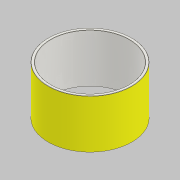
# Autodesk Inventor part: Stator Metal Ring
Saved by Autodesk Inventor 2020.1 (Build 241239000, 239)
## iProperties
Created: 2019-08-27
Part Number: Stator Metal Ring
Material: Steel, Wrought
Document SubType Name: Modeling
Designer: Oliver Frolovs
Density: 7.85 g/cm^3
Appearance: Steel
Mass: 2564.86 g
Surface Area: 1199.24 cm^2
Volume: 326.733 cm^3
Author: Oliver Frolovs
Autodesk Inventor part; units mm, degrees
ref_plane "YZ Plane" through (0, 0, 0) normal (1, 0, 0) x (0, 1, 0)
ref_plane "XZ Plane" through (0, 0, 0) normal (0, 1, 0) x (-1, 0, 0)
ref_plane "XY Plane" through (0, 0, 0) normal (0, 0, 1) x (1, 0, 0)
sketch "Sketch Metal Ring Profile" plane through (0, 0, 0) normal (0, 0, 1) x (1, 0, 0)
  circle A0 centre (0, 0) radius 89.75
  circle A1 centre (0, 0) radius 84
  dimension "d0" = 179.5
  dimension "d1" = 5.75
  constraints: 2 centre point, 1 coincident
  measures "d0" diameter of A0
  measures "d1" radial gap between concentric circles of A0 A1
extrude "Make Metal Ring by Extrusion of Its Profile" add sketch "Sketch Metal Ring Profile" along normal blind 104.1
chamfer "Chamfer1" distance 0.5 angle 45 2 edges at (-84, 0, 104.1) (-89.75, 0, 104.1)
equation "\"d0\" = PrototypeStatorMetalRingOuterDiameter"
equation "\"d1\" = PrototypeStatorMetalRingThickness"
equation "\"d2\" = PrototypeStatorMetalRingHeight"
equation "\"PrototypeStatorMetalRingOuterDiameter\" = 179.5"
equation "\"PrototypeStatorMetalRingThickness\" = 5.75"
equation "\"PrototypeStatorMetalRingHeight\" = 104.1"
body "Solid1"
